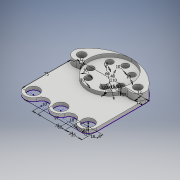
# Autodesk Inventor part: лаб2
Saved by Autodesk Inventor 2018 (Build 220112000, 112)
## iProperties
Created: 2020-04-07
Part Number: лаб2
Material: Типовые
Document SubType Name: Modeling
Designer: Nikita
Density: 1 g/cm^3
Appearance: По умолчанию
Author: Nikita
Autodesk Inventor part; units mm, degrees
ref_plane "YZ Plane" through (0, 0, 0) normal (1, 0, 0) x (0, 1, 0)
ref_plane "XZ Plane" through (0, 0, 0) normal (0, 1, 0) x (-1, 0, 0)
ref_plane "XY Plane" through (0, 0, 0) normal (0, 0, 1) x (1, 0, 0)
sketch "Эскиз1" plane through (0, 0, 0) normal (0, 0, 1) x (1, 0, 0)
  line L0 (0, 0) -> (110, 0) construction
  line L1 (110, 0) -> (55, 0) construction
  circle A0 centre (55, 0) radius 33
  line L2 (22, 0) -> (88, 0) construction
  line L3 (55, 0) -> (55, 33) construction
  line L4 (55, 0) -> (55, -33) construction
  circle A1 centre (55, 0) radius 24 construction
  circle A2 centre (55, 24) radius 5
  line L5 (55, 0) -> (71.9706, 16.9706) construction
  line L6 (71.9706, 16.9706) -> (38.0294, 16.9706) construction
  line L7 (55, 0) -> (38.0294, 16.9706) construction
  circle A3 centre (71.9706, 16.9706) radius 5
  circle A4 centre (38.0294, 16.9706) radius 5
  line L8 (55, 0) -> (78.1822, -6.2117) construction
  circle A5 centre (78.1822, -6.2117) radius 5
  line L9 (55, 0) -> (67.0003, -20.7844) construction
  circle A6 centre (67.0003, -20.7844) radius 5
  line L10 (55, 0) -> (42.9997, -20.7844) construction
  line L11 (78.1822, -6.2117) -> (31.8178, -6.2117) construction
  line L12 (31.8178, -6.2117) -> (55, 0) construction
  circle A7 centre (42.9997, -20.7844) radius 5
  circle A8 centre (31.8178, -6.2117) radius 5
  line L13 (0, 0) -> (12, 0) construction
  circle A9 centre (12, 0) radius 6
  line L14 (110, 0) -> (98, 0) construction
  circle A10 centre (98, 0) radius 6
  arc A11 (110, 0) -> (105.8455, 9.0801) centre (98, 0) ccw
  arc A12 (4.1545, 9.0801) -> (0, 0) centre (12, 0) ccw
  arc A13 (105.8455, 9.0801) -> (4.1545, 9.0801) centre (55, -33) ccw
  line L15 (0, 0) -> (0, -75)
  line L16 (0, -75) -> (110, -75) construction
  line L17 (110, -75) -> (110, 0)
  line L18 (55, 33) -> (55, -75) construction
  line L19 (110, -75) -> (97, -75) construction
  line L20 (0, -75) -> (13, -75) construction
  circle A14 centre (55, -75) radius 9
  circle A15 centre (13, -75) radius 9
  circle A16 centre (97, -75) radius 9
  line L21 (97, -75) -> (97, -88) construction
  line L22 (97, -88) -> (13, -88) construction
  line L23 (84, -75) -> (76, -75) construction
  line L24 (76, -75) -> (76, -84) construction
  arc A17 (85.6287, -81.3002) -> (110, -75) centre (97, -75) ccw
  arc A18 (85.6287, -81.3002) -> (66.3713, -81.3002) centre (76, -84) ccw
  arc A19 (43.6287, -81.3002) -> (66.3713, -81.3002) centre (55, -75) ccw
  line L25 (42, -75) -> (34, -75) construction
  line L26 (34, -75) -> (34, -84) construction
  line L27 (34, -84) -> (76, -84) construction
  arc A20 (43.6287, -81.3002) -> (24.3713, -81.3002) centre (34, -84) ccw
  arc A21 (0, -75) -> (24.3713, -81.3002) centre (13, -75) ccw
  arc A22 (0, 0) -> (15.9628, -11.3268) centre (12, 0) ccw
  arc A23 (25.7062, -15.1945) -> (15.9628, -11.3268) centre (18.6047, -18.878) ccw
  arc A24 (94.0372, -11.3268) -> (110, 0) centre (98, 0) ccw
  arc A25 (94.0372, -11.3268) -> (84.2938, -15.1945) centre (91.3953, -18.878) ccw
  dimension "d3" = 48
  dimension "d0" = 110
  dimension "d1" = 55
  dimension "d2" = 66
  dimension "d4" = 10
  dimension "d7" = 10
  dimension "d8" = 10
  dimension "d11" = 10
  dimension "d12" = 10
  dimension "d13" = 15
  dimension "d14" = 59.999
  dimension "d15" = 120.001
  dimension "d16" = 10
  dimension "d17" = 10
  dimension "d18" = 12
  dimension "d19" = 12
  dimension "d20" = 12
  dimension "d21" = 12
  dimension "d26" = 75
  dimension "d60" = 10
  dimension "d63" = 10
  dimension "d64" = 13
  dimension "d65" = 18
  dimension "d66" = 34
  dimension "d67" = 76
  dimension "d68" = 24.3713
  dimension "d69" = 26
  dimension "d70" = 9
  dimension "d71" = 68
  dimension "d72" = 97
  dimension "d77" = 8
  constraints: 54 end point, 31 point on circle, 25 centre point, 21 coincident, 11 tangent, 6 point on line, 5 vertical, 4 horizontal, 4 perpendicular, 1 concentric, 1 equal radius, 1 midpoint, 19 other
  measures "d0" distance of L0.start L0.end
  measures "d1" distance of L0.end L1.end
  measures "d2" diameter of A0
  measures "d4" diameter of A2
  measures "d7" diameter of A3
  measures "d8" diameter of A4
  measures "d11" diameter of A5
  measures "d12" diameter of A6
  measures "d13" angle of L8 L1
  measures "d14" angle of L1 L9
  measures "d15" angle of L1 L10
  measures "d16" diameter of A7
  measures "d17" diameter of A8
  measures "d18" distance of L0.start L13.end
  measures "d19" diameter of A9
  measures "d20" distance of L0.end L14.end
  measures "d21" diameter of A10
  measures "d26" distance of L0.start L15.end
  measures "d60" radius of A18
  measures "d63" radius of A20
  measures "d64" radius of A17
  measures "d65" diameter of A16
  measures "d66" distance between parallel lines of L24 L17
  measures "d67" distance between parallel lines of L26 L17
  measures "d68" distance from line of A17.start L17
  measures "d69" distance from line of L23.start L17
  measures "d71" distance from line of L25.start L17
  measures "d72" distance from line of L22.end L17
  measures "d77" radius of A23
extrude "Выдавливание1" add sketch "Эскиз1" along normal blind 10 contours A0
extrude "Выдавливание2" add sketch "Эскиз1" along normal blind 15 contours A23 A22 A12 A13 A0 | A0 A13 A11 A24 A25
extrude "Выдавливание3" add sketch "Эскиз1" along normal blind 5 contours A0 A25 A24 L17 A17 A18 A19 A20 A21 L15 A22 A23
